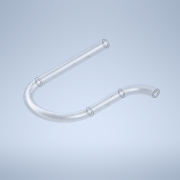
# Autodesk Inventor part: Hose
Saved by Autodesk Inventor 2020.2 (Build 242310000, 310)
## iProperties
Created: 2020-09-03
Part Number: Hose
Material: Generic
Document SubType Name: Modeling
Designer: JK
Density: 1 g/cm^3
Appearance: Water Bubbles
Author: JK
Autodesk Inventor part; units mm, degrees
ref_plane "YZ Plane" through (0, 0, 0) normal (1, 0, 0) x (0, 1, 0)
ref_plane "XZ Plane" through (0, 0, 0) normal (0, 1, 0) x (-1, 0, 0)
sketch "Sketch1" plane through (0, 0, 0) normal (0, 1, 0) x (-1, 0, 0)
  arc A0 (14.5, 0) -> (-14.5, 0) centre (0, 0) ccw
  line L0 (14.5, 0) -> (14.5, -18)
  line L1 (-14.5, 0) -> (-14.5, -18)
  dimension "d0" = 29
  dimension "d9" = 18
  constraints: 4 end point, 2 point on circle, 2 vertical, 1 centre point, 1 coincident, 1 horizontal alignment, 1 point on line
  measures "d0" diameter of A0
  measures "d9" distance of L0.start L0.end
ref_plane "Work Plane1" through (-14.5, 0, -18) normal (0, 0, 1) x (1, 0, 0)
sketch "Sketch2" plane through (-14.5, 0, -18) normal (0, 0, 1) x (1, 0, 0)
  circle A0 centre (0, 0) radius 2
  circle A1 centre (0, 0) radius 1.25
  point P0 (14.5, 0)
  dimension "d1" = 4
  dimension "d2" = 2.5
  constraints: 2 centre point, 1 coincident
  measures "d1" diameter of A0
  measures "d2" diameter of A1
sweep "Sweep1" add profiles "Sketch2" path "Sketch1" path curves L0 A0
sketch "Sketch3" plane through (14.5, 0, 0) normal (0, 0, -1) x (-1, 0, 0)
  circle A0 centre (0, 0) radius 1.25 projected
  circle A1 centre (0, 0) radius 2 projected
  point P0 (14.5, 0)
extrude "Extrusion1" add sketch "Sketch3" along normal up to surface (18 mm away)
sketch "Sketch5" plane through (14.5, 0, -18) normal (0, 0, -1) x (-1, 0, 0)
  line L0 (-9.7666, -8.325) -> (-9.7666, 9.6914)
  circle A0 centre (0, 0) radius 1.25 projected
  circle A1 centre (0, 0) radius 2 projected
  point P0 (14.5, 0)
  constraints: 2 end point, 1 vertical
revolve "Revolution2" add sketch "Sketch5" angle 90 about axis through (24.2666, -8.325, -18) along (0, -1, 0)
sketch "Sketch6" plane through (-14.5, 0, -18) normal (0, 0, -1) x (-1, 0, 0)
  circle A0 centre (0, 0) radius 1.25 projected
  circle A1 centre (0, 0) radius 2 projected
  point P0 (-14.5, 0)
extrude "Extrusion2" add sketch "Sketch6" along normal blind 20
body "Solid1"
